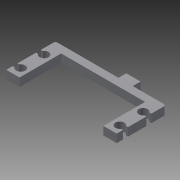
# Autodesk Inventor part: MG996RBracketTop
Saved by Autodesk Inventor 2014 SP1 (Build 180222100, 222)
## iProperties
Created: 2017-02-23
Part Number: MG996RBracketTop
Material: Generic
Document SubType Name: Modeling
Designer: danielsikar
Density: 1 g/cm^3
Appearance: Default
Author: danielsikar
Autodesk Inventor part; units mm, degrees
ref_plane "YZ Plane" through (0, 0, 0) normal (1, 0, 0) x (0, 1, 0)
sketch "Sketch1" plane through (0, 0, 0) normal (0, 0, 1) x (1, 0, 0)
  line L0 (5.8439, -14.5) -> (6.8, -14.5) projected
  line L1 (6.8, -5.5) -> (6.8, -14.5) projected
  line L2 (6.8, -5.5) -> (5.8439, -5.5) projected
  arc A0 (5.8439, -3.1) -> (5.8439, -5.5) centre (4, -4.3) ccw projected
  line L3 (5.8439, -3.1) -> (6.8, -3.1) projected
  line L4 (6.8, 0) -> (6.8, -3.1) projected
  line L5 (0, 0) -> (6.8, 0) projected
  line L6 (0, -20) -> (0, 0) projected
  line L7 (0, -20) -> (6.8, -20) projected
  line L8 (6.8, -16.9) -> (6.8, -20) projected
  line L9 (6.8, -16.9) -> (5.8439, -16.9) projected
  arc A1 (5.8439, -14.5) -> (5.8439, -16.9) centre (4, -15.7) ccw projected
  line L10 (-47.1, -14.5) -> (-46.1439, -14.5) projected
  arc A2 (-46.1439, -16.9) -> (-46.1439, -14.5) centre (-44.3, -15.7) ccw projected
  line L11 (-46.1439, -16.9) -> (-47.1, -16.9) projected
  line L12 (-47.1, -16.9) -> (-47.1, -20) projected
  line L13 (-40.3, -20) -> (-47.1, -20) projected
  line L14 (-40.3, 0) -> (-40.3, -20) projected
  line L15 (-40.3, 0) -> (-47.1, 0) projected
  line L16 (-47.1, 0) -> (-47.1, -3.1) projected
  line L17 (-47.1, -3.1) -> (-46.1439, -3.1) projected
  arc A3 (-46.1439, -5.5) -> (-46.1439, -3.1) centre (-44.3, -4.3) ccw projected
  line L18 (-46.1439, -5.5) -> (-47.1, -5.5) projected
  line L19 (-47.1, -5.5) -> (-47.1, -14.5) projected
extrude "Extrusion1" add sketch "Sketch1" along normal blind 4
sketch "Sketch2" plane through (0, 0, 0) normal (0, 1, 0) x (1, 0, 0)
  line L0 (0, 0) -> (6.8, 0) projected
  line L1 (0, 0) -> (0, -4) projected
  line L2 (6.8, -4) -> (0, -4) projected
  line L3 (6.8, 0) -> (6.8, -4) projected
  line L4 (-47.1, 0) -> (-47.1, -4) projected
  line L5 (-40.3, -4) -> (-47.1, -4) projected
  line L6 (6.8, 0) -> (-47.1, 0)
  line L7 (-47.1, 0) -> (-47.1, -4)
  line L8 (-47.1, -4) -> (6.8, -4)
  line L9 (6.8, -4) -> (6.8, 0)
  constraints: 8 end point, 2 parallel, 1 horizontal, 1 perpendicular
extrude "Extrusion2" add sketch "Sketch2" along normal blind 4 contours L1 L8 L5 L4 L6
sketch "Sketch3" plane through (0, 0, 4) normal (1, 0, 0) x (0, 0, -1)
  line L0 (4, 0) -> (0, 0) projected
  line L1 (4, 4) -> (4, 0) projected
  line L2 (0, 4) -> (4, 4) projected
  line L3 (0, 0) -> (0, 4) projected
extrude "Extrusion3" add sketch "Sketch3" along normal up to surface (6.8 mm away)
sketch "Sketch4" plane through (0, 4, 0) normal (0, 1, 0) x (1, 0, 0)
  line L0 (6.8, 0) -> (-47.1, 0) projected
  line L1 (-47.1, -4) -> (6.8, -4) projected
  line L2 (-9.3767, -8.1) -> (-9.3767, -13.1) construction
  line L3 (-21.8189, -8.1) -> (-9.3767, -8.1) construction
  arc A0 (-17.3767, -8.1) -> (-40.8, 16.4941) centre (-48.3, -14.1) ccw construction
  line L4 (-9.3767, -4) -> (-16.3767, -4) construction
  line L5 (-16.3767, -4) -> (-16.3767, -8.1) construction
  line L6 (-16.3767, -8.1) -> (-9.3767, -8.1) construction
  line L7 (-9.3767, -8.1) -> (-9.3767, -4) construction
  line L8 (-9.3767, -4) -> (-16.3767, -4)
  line L9 (-16.3767, -4) -> (-16.3767, 0)
  line L10 (-16.3767, 0) -> (-9.3767, 0)
  line L11 (-9.3767, 0) -> (-9.3767, -4)
  point P0 (0, 0)
  dimension "d6" = 7
  constraints: 16 end point, 4 parallel, 3 point on line, 2 horizontal, 2 perpendicular
  measures "d6" distance of L6.end L5.end
ref_plane "Work Plane1" through (-21.8189, 29, 8.1) normal (0, 1, 0) x (0, 0, 1)
extrude "Extrusion4" add sketch "Sketch4" along normal up to surface (25 mm away)
sketch "Sketch5" plane through (0, 0, 4) normal (0, 0, 1) x (1, 0, 0)
  circle A0 centre (-13.3767, 24) radius 2 construction
  line L0 (-21.8189, 24) -> (-17.3767, 24) construction
  line L1 (-21.8189, 24) -> (-21.8189, 29) construction
  line L2 (-21.8189, 29) -> (-9.3767, 29) construction
  line L3 (-9.3767, 19) -> (-9.3767, 29) construction
  line L4 (-17.3767, 19) -> (-9.3767, 19) construction
  line L5 (-17.3767, 24) -> (-17.3767, 19) construction
  line L6 (-9.3767, 19) -> (-16.3767, 19) construction
  line L7 (-16.3767, 19) -> (-16.3767, 29) construction
  line L8 (-16.3767, 29) -> (-9.3767, 29) construction
  line L9 (-9.3767, 29) -> (-9.3767, 19) construction
  line L10 (-9.3767, 19) -> (-16.3767, 19)
  line L11 (-16.3767, 19) -> (-16.3767, 29)
  line L12 (-16.3767, 29) -> (-9.3767, 29)
  line L13 (-9.3767, 29) -> (-9.3767, 19)
  circle A1 centre (-13.3767, 24) radius 2
  constraints: 16 end point, 4 parallel, 2 horizontal, 2 perpendicular, 1 centre point, 1 coincident, 1 concentric
ref_plane "Work Plane2" through (-21.8189, 19, 8.1) normal (0, 0, -1) x (0, 1, 0)
extrude "Extrusion5" add sketch "Sketch5" along normal up to surface (4.1 mm away)
sketch "Sketch6" plane through (-16.3767, 19, 8.1) normal (-1, 0, 0) x (0, 0, 1)
  line L0 (0, 5) -> (-24.5941, 5) construction
  line L1 (0, 0) -> (-24.5941, 0) construction
  line L2 (-8.1, 10) -> (0.5132, 10) construction
  line L3 (0.5132, 10) -> (0.5132, 5) construction
  line L4 (0.5132, 5) -> (-8.1, 5) construction
  line L5 (-8.1, 5) -> (-8.1, 10) construction
  line L6 (-8.1, 10) -> (0, 10)
  line L7 (0, 10) -> (0, 5)
  line L8 (0, 5) -> (-8.1, 5)
  line L9 (-8.1, 5) -> (-8.1, 10)
  point P0 (-8.1, -19)
  constraints: 16 end point, 4 parallel, 2 horizontal, 2 perpendicular
extrude "Extrusion6" add sketch "Sketch6" along normal blind 5
sketch "Sketch7" plane through (-16.3767, 24, 0) normal (0, -1, 0) x (1, 0, 0)
  line L0 (0, 8.1) -> (0, 0) projected
  line L1 (0, 8.1) -> (-5, 8.1) projected
  line L2 (-5, 0) -> (-5, 8.1) projected
  line L3 (0, 0) -> (-5, 0) projected
  point P0 (16.3767, 0)
extrude "Extrusion7" cut sketch "Sketch7" against normal blind 0.4
sketch "Sketch8" plane through (0, 0, 0) normal (0, 0, -1) x (-1, 0, 0)
  circle A0 centre (13.3767, 24) radius 2 construction
  circle A1 centre (13.3767, 24) radius 2 projected
extrude "Extrusion8" cut sketch "Sketch8" against normal blind 4
fillet "Fillet3" radius 1 1 edges at (-16.3767, 24.4, 4.05)
sketch "Sketch9" plane through (-9.3767, 19, 8.1) normal (1, 0, 0) x (0, 0, -1)
  line L0 (0, 0) -> (0, 10) projected
  line L1 (8.1, 7) -> (0, 7) construction
  line L2 (8.1, 3) -> (0, 3) construction
  line L3 (24.5941, 5) -> (0, 5) construction
  line L4 (-5, 5) -> (0, 5) construction
  line L5 (4, 8.75) -> (7.5, 8.75)
  line L6 (7.5, 8.75) -> (7.5, 1.25)
  line L7 (7.5, 1.25) -> (4, 1.25)
  line L8 (4, 1.25) -> (4, 8.75)
  point P0 (8.1, -19)
  point P1 (4, 5)
  dimension "d20" = 3.5
  dimension "d21" = 7.5
  dimension "d22" = 4
  constraints: 8 end point, 2 parallel, 1 horizontal, 1 midpoint, 1 perpendicular, 1 point on line
  measures "d20" distance of L6.end L7.end
  measures "d21" distance of L5.end L6.end
  measures "d22" distance between parallel lines of L0 L8
extrude "Extrusion9" cut sketch "Sketch9" against normal blind 7.5
sketch "Sketch10" plane through (-16.3767, 19, 4) normal (0, -1, 0) x (1, 0, 0)
  line L0 (0, 4.1) -> (7, 4.1) projected
  line L1 (0, 0) -> (0, 4.1) projected
  line L2 (7, 0) -> (0, 0) projected
  line L3 (7, 0) -> (7, 4.1) projected
  point P0 (16.3767, -4)
extrude "Extrusion10" add sketch "Sketch10" along normal blind 3
fillet "Fillet4" radius 3 1 edges at (-12.8767, 16, 4)
sketch "Sketch11" plane through (0, 0, 0) normal (0, -1, 0) x (1, 0, 0)
  line L0 (-40.3, 0) -> (-40.3, 4) projected
  line L1 (0, 0) -> (-40.3, 0) projected
  line L2 (0, 0) -> (0, 4) projected
  line L3 (-40.3, 4) -> (0, 4) projected
extrude "Extrusion11" cut sketch "Sketch11" against normal blind 0.3
sketch "Sketch12" plane through (0, -20, 0) normal (-1, 0, 0) x (0, 0, 1)
  line L0 (0, 0) -> (0, 20.3) projected
  line L1 (0, 0) -> (4, 0) projected
  line L2 (4, 20.3) -> (4, 0) projected
  line L3 (4, 20.3) -> (0, 20.3) projected
  point P0 (0, 20)
extrude "Extrusion12" cut sketch "Sketch12" against normal blind 0.3
sketch "Sketch13" plane through (-40.3, -20, 4) normal (1, 0, 0) x (0, 0, -1)
  line L0 (4, 0) -> (4, 20.3) projected
  line L1 (4, 20.3) -> (0, 20.3) projected
  line L2 (0, 0) -> (0, 20.3) projected
  line L3 (4, 0) -> (0, 0) projected
  point P0 (4, 20)
extrude "Extrusion13" cut sketch "Sketch13" against normal blind 0.3
fillet "Fillet5" radius 1 2 edges at (6.8, 4, 2) (-47.1, 4, 2)
sketch "Sketch15" plane through (0, 0, 0) normal (0, 0, -1) x (-1, 0, 0)
  circle A0 centre (13.3767, 24) radius 2 projected
  line L0 (9.3767, 29) -> (21.3767, 29)
  line L1 (21.3767, 29) -> (21.3767, 7.8113)
  line L2 (21.3767, 7.8113) -> (9.3767, 7.8113)
  line L3 (9.3767, 7.8113) -> (9.3767, 29)
  point P0 (0, 0)
  constraints: 8 end point, 2 parallel, 1 horizontal, 1 perpendicular
extrude "Extrusion14" cut sketch "Sketch15" against normal through all
body "Solid1"
